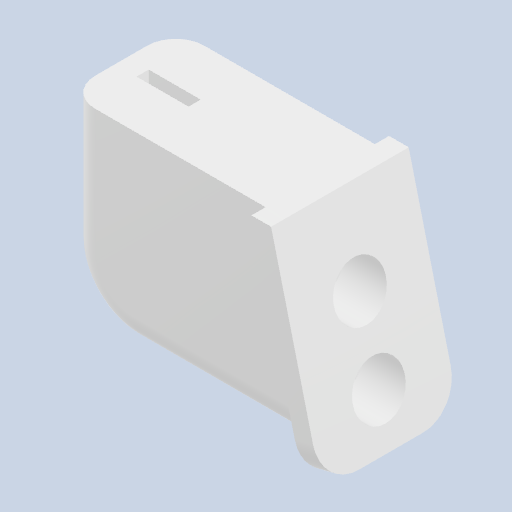
# Autodesk Inventor part: buton
Saved by Autodesk Inventor 2024 (Build 280153000, 153)
## iProperties
Created: 2024-04-18
Part Number: buton
Material: PBT Plastic
Document SubType Name: Modeling
Designer: mirun
Density: 1.31 g/cm^3
Appearance: Smooth - White
Author: mirun
Autodesk Inventor part; units mm, degrees
ref_plane "YZ Plane" through (0, 0, 0) normal (1, 0, 0) x (0, 1, 0)
sketch "Sketch1" plane through (0, 0, 0) normal (1, 0, 0) x (0, 1, 0)
  line L0 (-10, 5.75) -> (10, 5.75)
  line L1 (10, 5.75) -> (10, -5.75)
  line L2 (10, -5.75) -> (-10, -5.75)
  line L3 (-10, -5.75) -> (-10, 5.75)
  line L4 (-10, 5.75) -> (10, -5.75) construction
  line L5 (10, 5.75) -> (-10, -5.75) construction
  point P0 (0, 0)
  dimension "d0" = 20
  dimension "d1" = 11.5
  constraints: 12 end point, 2 midpoint, 2 parallel, 1 horizontal, 1 perpendicular
  measures "d0" distance of L1.end L2.end
  measures "d1" distance of L0.end L1.end
extrude "Extrusion1" add sketch "Sketch1" along normal blind 21
ref_plane "Work Plane1" through (21, 10, -5.75) normal (0.9701266, 0.2425992, 0) x (0, 0, 1)
sketch "Sketch2" plane through (0, 10, 5.75) normal (0, 1, 0) x (1, 0, 0)
  line L0 (7.75, 5.1) -> (2.25, 5.1)
  line L1 (2.25, 5.1) -> (2.25, 6.4)
  line L2 (2.25, 6.4) -> (7.75, 6.4)
  line L3 (7.75, 6.4) -> (7.75, 5.1)
  line L4 (7.75, 5.1) -> (2.25, 6.4) construction
  line L5 (2.25, 5.1) -> (7.75, 6.4) construction
  line L6 (7.25, 5.1) -> (2.75, 5.1)
  line L7 (2.75, 5.1) -> (2.75, 6.4)
  line L8 (2.75, 6.4) -> (7.25, 6.4)
  line L9 (7.25, 6.4) -> (7.25, 5.1)
  line L10 (7.25, 5.1) -> (2.75, 6.4) construction
  line L11 (2.75, 5.1) -> (7.25, 6.4) construction
  line L12 (0, 11.5) -> (0, 0) construction
  point P0 (0, 5.75)
  point P1 (5, 5.75)
  point P2 (5, 5.75)
  point P3 (7.25, 5.1)
  point P4 (2.75, 5.1)
  point P5 (0, 5.75)
  dimension "d4" = 5.5
  dimension "d5" = 1.3
  dimension "d6" = 4.5
  dimension "d20" = 5
  constraints: 24 end point, 6 midpoint, 4 parallel, 2 horizontal, 2 perpendicular, 1 horizontal alignment, 1 point on line
  measures "d4" distance of L1.end L2.end
  measures "d5" distance of L0.end L1.end
  measures "d6" distance of L7.end L8.end
  measures "d20" distance from line of L12 point (5, 5.75)
extrude "Extrusion2" cut sketch "Sketch2" against normal blind 10
extrude "Extrusion3" cut sketch "Sketch2" against normal blind 14 contours L0 L7 L2 L9
fillet "Fillet1" radius 3 4 edges at (0, 0, 5.75) (10.5, -10, 5.75) (10.5, -10, -5.75) (0, 0, -5.75)
fillet "Fillet2" radius 7 3 edges at (0.8787, -9.1213, -4.8713) (0.8787, -9.1213, 4.8713) (0, -10, 0)
sketch "Sketch4" plane through (21, 0, 0) normal (1, 0, 0) x (0, 0, -1)
  arc A0 (2.75, -10) -> (5.75, -7) centre (2.75, -7) ccw projected
  line L0 (5.75, -7) -> (5.75, 10) projected
  line L1 (5.75, 10) -> (-5.75, 10) projected
  line L2 (-5.75, 10) -> (-5.75, -7) projected
  arc A1 (-5.75, -7) -> (-2.75, -10) centre (-2.75, -7) ccw projected
  line L3 (-2.75, -10) -> (2.75, -10) projected
  point P0 (0, 0)
extrude "Extrusion5" add sketch "Sketch4" along normal up to surface surface through (21, 10, -5.75) normal (0.9701266, 0.2425992, 0)
sketch "Sketch6" plane through (21, 10, 5.75) normal (0.9701266, 0.2425992, 0) x (0, 0, -1)
  line L0 (11.5, 0) -> (11.5, -17.5235) projected
  line L1 (11.5, 0) -> (0, 0) projected
  line L2 (0, -17.5235) -> (0, 0) projected
  line L3 (8.5, -20.6159) -> (3, -20.6159) projected
  line L4 (-1.5, 0) -> (13, 0)
  line L5 (13, 0) -> (13, -18.7739)
  line L6 (9.158, -22.6159) -> (2.342, -22.6159)
  line L7 (-1.5, -18.7739) -> (-1.5, 0)
  arc A0 (-1.5, -18.7739) -> (2.342, -22.6159) centre (2.342, -18.7739) ccw
  arc A1 (9.158, -22.6159) -> (13, -18.7739) centre (9.158, -18.7739) ccw
  point P0 (5.75, -4.6067)
  dimension "d21" = 1.5
  dimension "d22" = 1.5
  dimension "d23" = 2
  dimension "d24" = 3.842
  constraints: 8 end point, 4 point on circle, 4 tangent, 2 centre point, 2 parallel, 1 equal radius, 1 horizontal, 1 perpendicular
  measures "d21" distance between parallel lines of L7 L2
  measures "d22" distance between parallel lines of L5 L0
  measures "d23" distance between parallel lines of L6 L3
  measures "d24" radius of A0
extrude "Extrusion6" add sketch "Sketch6" along normal blind 2
sketch "Sketch7" plane through (0, 0, 0) normal (-1, 0, 0) x (0, 0, 1)
  line L0 (7.25, 10.4852) -> (7.25, -7.7278) construction
  line L1 (-7.6184, 10) -> (7.25, 10)
  line L2 (7.25, 10) -> (7.25, 10.4852)
  line L3 (7.25, 10.4852) -> (-7.6184, 10.4852)
  line L4 (-7.6184, 10.4852) -> (-7.6184, 10)
  line L5 (3.408, -11.4551) -> (-3.408, -11.4551) construction
  line L6 (-3.408, -11.4551) -> (7.25, -11.4551)
  line L7 (7.25, -11.4551) -> (7.25, -13.162)
  line L8 (7.25, -13.162) -> (-3.408, -13.162)
  line L9 (-3.408, -13.162) -> (-3.408, -11.4551)
  line L10 (-3.408, -11.4551) -> (-7.4388, -11.4551)
  line L11 (-7.4388, -11.4551) -> (-7.4388, -13.1256)
  line L12 (-7.4388, -13.1256) -> (-3.408, -13.1256)
  line L13 (-3.408, -13.1256) -> (-3.408, -11.4551)
  point P0 (0, 0)
  point P1 (-2.75, 10)
  constraints: 24 end point, 6 parallel, 3 horizontal, 3 perpendicular, 2 point on line
extrude "Extrusion7" cut sketch "Sketch7" against normal through all
ref_plane "Work Plane2" through (28.427, 0, 0) normal (-1, 0, 0) x (0, 0, 1)
sketch "Sketch8" plane through (28.427, 0, 0) normal (-1, 0, 0) x (0, 0, 1)
  circle A0 centre (0, 1.5449) radius 2.75
  circle A1 centre (0, -6.4551) radius 2.75
  line L0 (3.408, -11.4551) -> (-3.408, -11.4551) construction
  point P0 (0, 0)
  dimension "d30" = 5.5
  dimension "d31" = 5.5
  dimension "d36" = 8
  dimension "d37" = 5
  constraints: 2 centre point, 2 vertical alignment
  measures "d30" diameter of A0
  measures "d31" diameter of A1
  measures "d36" distance of A1.centre A0.centre
  measures "d37" distance from line of L0 A1.centre
extrude "Extrusion8" cut sketch "Sketch8" along normal blind 5.5 contours A1
extrude "Extrusion9" cut sketch "Sketch8" along normal blind 7.5 contours A0
body "Solid1"
